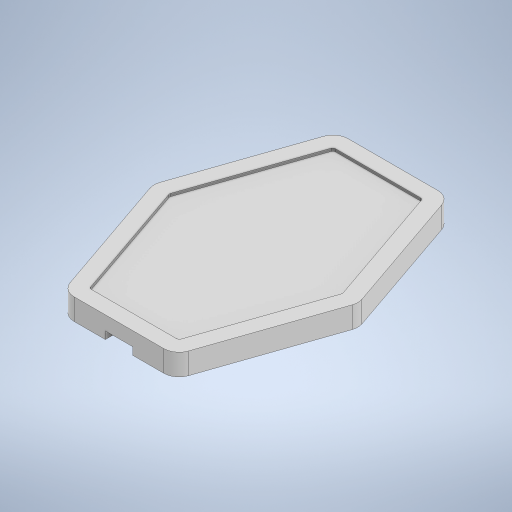
# Autodesk Inventor part: Part1
Saved by Autodesk Inventor 2023.1 (Build 271208000, 208)
## iProperties
Created: 2022-10-21
Part Number: Part1
Material: Generic
Document SubType Name: Modeling
Designer: jshin23
Density: 1 g/cm^3
Appearance: Default
Author: jshin23
Autodesk Inventor part; units mm, degrees
ref_plane "YZ Plane" through (0, 0, 0) normal (1, 0, 0) x (0, 1, 0)
ref_plane "XZ Plane" through (0, 0, 0) normal (0, 1, 0) x (-1, 0, 0)
ref_plane "XY Plane" through (0, 0, 0) normal (0, 0, 1) x (1, 0, 0)
sketch "Sketch1" plane through (0, 0, 0) normal (0, 1, 0) x (-1, 0, 0)
  line L0 (94.0269, 81.28) -> (27.9869, 81.28)
  line L1 (94.0269, -81.28) -> (27.9869, -81.28)
  line L2 (94.0269, 81.28) -> (122.0139, 0)
  line L3 (94.0269, 81.28) -> (179.9904, 81.28) construction
  line L4 (122.0139, 0) -> (94.0269, -81.28)
  line L5 (27.9869, 81.28) -> (0, 0)
  line L6 (27.9869, 81.28) -> (113.9504, 81.28) construction
  line L7 (0, 0) -> (27.9869, -81.28)
  dimension "d6" = 66.04
  dimension "d7" = 162.56
  dimension "d8" = 71
  dimension "d9" = 109
  dimension "d10" = 109
  constraints: 16 end point, 5 equal length, 4 horizontal, 1 coincident
  measures "d6" distance of L0.start L0.end
  measures "d7" distance between parallel lines of L0 L1
  measures "d8" angle of L2 L3
  measures "d9" angle of L5 L6
  measures "d10" angle of L7 L1
extrude "Extrusion1" add sketch "Sketch1" along normal blind 12.7
fillet "Fillet1" radius 8.89 6 edges at (-27.9869, 6.35, 81.28) (-94.0269, 6.35, 81.28) (0, 6.35, 0) (-27.9869, 6.35, -81.28) (-122.0139, 6.35, 0) (-94.0269, 6.35, -81.28)
sketch "Sketch3" plane through (0, 12.7, 0) normal (0, 1, 0) x (1, 0, 0)
  line L0 (-35.7374, 72.39) -> (-86.2503, 72.39)
  line L1 (-35.7374, -72.39) -> (-86.2503, -72.39)
  line L2 (-34.2004, 71.2936) -> (-9.8342, 0.5292)
  line L3 (-34.5779, 72.39) -> (40.264, 72.39) construction
  line L4 (-9.8342, -0.5292) -> (-34.2004, -71.2936)
  line L5 (-87.7874, 71.2936) -> (-112.1535, 0.5292)
  line L6 (-87.4099, 72.39) -> (-12.568, 72.39) construction
  line L7 (-112.1535, -0.5292) -> (-87.7874, -71.2936)
  arc A0 (-86.2503, 72.39) -> (-87.7874, 71.2936) centre (-86.2503, 70.7644) ccw
  arc A1 (-112.1535, 0.5292) -> (-112.1535, -0.5292) centre (-110.6165, 0) ccw
  arc A2 (-87.7874, -71.2936) -> (-86.2503, -72.39) centre (-86.2503, -70.7644) ccw
  arc A3 (-35.7374, -72.39) -> (-34.2004, -71.2936) centre (-35.7374, -70.7644) ccw
  arc A4 (-9.8342, -0.5292) -> (-9.8342, 0.5292) centre (-11.3713, 0) ccw
  arc A5 (-34.2004, 71.2936) -> (-35.7374, 72.39) centre (-35.7374, 70.7644) ccw
  point P0 (0, 0)
  point P1 (-112.3358, 0)
  point P2 (-34.5779, -72.39)
  point P3 (-87.4099, -72.39)
  point P4 (-9.652, 0)
  point P5 (-112.3358, 0)
  dimension "d18" = 52.832
  dimension "d19" = 144.78
  dimension "d20" = 71
  dimension "d21" = 109
  dimension "d22" = 109
  dimension "d23" = 9.652
  dimension "d24" = 0
  dimension "d27" = 1.6256
  constraints: 16 end point, 12 point on circle, 12 point on line, 12 tangent, 6 centre point, 5 equal length, 5 equal radius, 4 horizontal, 1 coincident
  measures "d18" distance of L3.start L6.start
  measures "d19" distance between parallel lines of L0 L1
  measures "d20" angle of L2 L3
  measures "d21" angle of L5 L6
  measures "d22" angle of L7 L1
  measures "d23" distance of point (-9.652, 0) point (0, 0)
  measures "d24" vertical distance of point (0, 0) point (-9.652, 0)
  measures "d27" radius of A0
extrude "Extrusion3" cut sketch "Sketch3" against normal blind 1.6256
sketch "Sketch4" plane through (0, 0, 0) normal (0, -1, 0) x (1, 0, 0)
  line L0 (-52.8789, 81.28) -> (-69.1349, 81.28)
  line L1 (-69.1349, 81.28) -> (-69.1349, 64.135)
  line L2 (-65.9599, 60.96) -> (-56.0539, 60.96)
  line L3 (-52.8789, 64.135) -> (-52.8789, 81.28)
  line L4 (-87.6858, 81.28) -> (-34.3281, 81.28) projected
  arc A0 (-56.0539, 60.96) -> (-52.8789, 64.135) centre (-56.0539, 64.135) ccw
  arc A1 (-69.1349, 64.135) -> (-65.9599, 60.96) centre (-65.9599, 64.135) ccw
  point P0 (0, 0)
  point P1 (-69.1349, 60.96)
  point P2 (-52.8789, 60.96)
  point P3 (-61.0069, 81.28)
  dimension "d28" = 16.256
  dimension "d29" = 20.32
  dimension "d32" = 3.175
  constraints: 8 end point, 4 point on circle, 4 point on line, 4 tangent, 2 centre point, 2 midpoint, 2 parallel, 1 equal radius, 1 horizontal, 1 perpendicular
  measures "d28" distance of point (-52.879, 60.96) point (-69.135, 60.96)
  measures "d29" distance of point (-52.879, 60.96) L0.start
  measures "d32" radius of A0
extrude "Extrusion4" cut sketch "Sketch4" against normal blind 4.445
mirror "Mirror2" about plane through (0, 0, 0) normal (0, 0, 1) of "Extrusion4"
body "Solid1"
